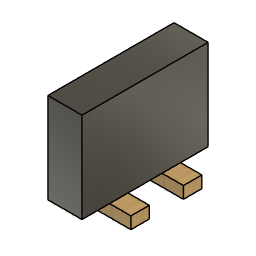
Computer-V1 (Autodesk Fusion 360 design; units mm, degrees)
Autodesk Fusion 360 part; units mm, degrees
sketch "Skizze1" plane through (0, 0, 0) normal (0, 0, 1) x (1, 0, 0)
  line L0 (-250, 20) -> (-25, 20)
  line L1 (-25, 20) -> (-25, -34)
  line L2 (-25, -34) -> (-250, -34)
  line L3 (-250, -34) -> (-250, 20)
  line L4 (-250, 20) -> (-25, 20)
  line L5 (-25, -34) -> (-250, -34)
  line L6 (-250, -34) -> (-250, 20)
  line L7 (-25, 20) -> (-25, -34)
  line L8 (-25, -188) -> (-250, -188)
  line L9 (-25, -134) -> (-25, -188)
  line L10 (-250, -188) -> (-250, -134)
  line L11 (-250, -134) -> (-25, -134)
  dimension "d3" = 225
  dimension "d4" = 54
  dimension "d5" = 225
  dimension "d6" = 54
  dimension "d9" = 225
  dimension "d10" = 54
  dimension "d11" = 100
  constraint horizontal L0
  constraint vertical L1
  constraint horizontal L2
  constraint vertical L3
  constraint horizontal L4
  constraint vertical L7
  constraint horizontal L5
  constraint vertical L6
  constraint horizontal L11
  constraint vertical L9
  constraint horizontal L8
  constraint vertical L10
  measures "d3" distance of L0.start L0.end
  measures "d4" distance of L0.start L2.end
  measures "d5" distance of L0.end L0.start
  measures "d6" distance of L0.start L2.end
  measures "d9" distance of L10.end L9.start
  measures "d10" distance of L10.end L8.end
  measures "d11" distance of L5 L11
extrude "Extrusion1" add sketch "Skizze1" along normal blind 35 makes body 1 at (-175, 2, 0) makes body 2 at (-100, -170, 0)
sketch "Skizze2" plane through (0, 0, 35) normal (0, 0, 1) x (-1, 0, 0)
  line L0 (25, -20) -> (250, -20)
  line L1 (250, -20) -> (250, 34)
  line L2 (250, 34) -> (25, 34)
  line L3 (25, 34) -> (25, -20)
  line L4 (187.5, -101) -> (87.5, -101)
  line L5 (87.5, -101) -> (87.5, 269)
  line L6 (87.5, 269) -> (187.5, 269)
  line L7 (187.5, 269) -> (187.5, -101)
  line L8 (25, 134) -> (25, 188)
  line L9 (250, 188) -> (250, 134)
  line L10 (25, 188) -> (250, 188)
  line L11 (250, -20) -> (25, -20)
  dimension "d14" = 100
  dimension "d15" = 370
  dimension "d18" = 81
  dimension "d19" = 81
  dimension "d20" = 62.5
  dimension "d21" = 62.5
  constraint horizontal L4
  constraint vertical L5
  constraint horizontal L6
  constraint vertical L7
  measures "d14" distance of L4.start L4.end
  measures "d15" distance of L4.start L6.end
  measures "d18" distance of L6 L10
  measures "d19" distance of L4 L11
  measures "d20" distance of L7 L9
  measures "d21" distance of L5 L8
extrude "Extrusion2" add sketch "Skizze2" along normal blind 265 separate body contours L0 L2 L5 L7 L11 | L0 L4 L5 L7 L11 | L2 L5 L7 L10 | L5 L6 L7 L10 makes body 3
named bodies: "Bodenabstand-2", "Bodenabstand-1", "PC"
